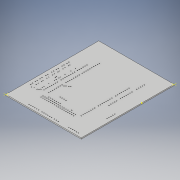
# Autodesk Inventor part: board
Saved by Autodesk Inventor 2019 (Build 230136000, 136)
## iProperties
Created: 2020-01-04
Part Number: board
Material: Типовые
Document SubType Name: Modeling
Designer: Петров Иван
Density: 1 g/cm^3
Appearance: По умолчанию
Author: Петров Иван
Autodesk Inventor part; units mm, degrees
ref_plane "YZ Plane" through (0, 0, 0) normal (1, 0, 0) x (0, 1, 0)
ref_plane "XZ Plane" through (0, 0, 0) normal (0, 1, 0) x (-1, 0, 0)
ref_plane "XY Plane" through (0, 0, 0) normal (0, 0, 1) x (1, 0, 0)
sketch "Эскиз1" plane through (0, 0, 0) normal (0, 1, 0) x (-1, 0, 0)
  circle A0 centre (25.4, 31.75) radius 0.508
  circle A1 centre (91.44, 17.78) radius 0.4064
  circle A2 centre (83.82, 45.72) radius 0.4064
  circle A3 centre (91.44, 45.72) radius 0.4064
  circle A4 centre (83.82, 3.81) radius 0.4064
  circle A5 centre (25.4, 39.37) radius 0.508
  circle A6 centre (25.4, 41.91) radius 0.508
  circle A7 centre (25.4, 44.45) radius 0.508
  circle A8 centre (25.4, 46.99) radius 0.508
  circle A9 centre (25.4, 49.53) radius 0.508
  circle A10 centre (25.4, 52.07) radius 0.508
  circle A11 centre (25.4, 54.61) radius 0.508
  circle A12 centre (25.4, 36.83) radius 0.508
  circle A13 centre (73.66, 34.29) radius 0.508
  circle A14 centre (73.66, 36.83) radius 0.508
  circle A15 centre (73.66, 39.37) radius 0.508
  circle A16 centre (73.66, 41.91) radius 0.508
  circle A17 centre (73.66, 44.45) radius 0.508
  circle A18 centre (73.66, 46.99) radius 0.508
  circle A19 centre (73.66, 49.53) radius 0.508
  circle A20 centre (73.66, 31.75) radius 0.508
  circle A21 centre (25.4, 16.51) radius 0.508
  circle A22 centre (25.4, 19.05) radius 0.508
  circle A23 centre (25.4, 21.59) radius 0.508
  circle A24 centre (25.4, 24.13) radius 0.508
  circle A25 centre (25.4, 26.67) radius 0.508
  circle A26 centre (25.4, 29.21) radius 0.508
  circle A27 centre (63.5, 57.15) radius 0.508
  circle A28 centre (25.4, 13.97) radius 0.508
  circle A29 centre (73.66, 11.43) radius 0.508
  circle A30 centre (73.66, 13.97) radius 0.508
  circle A31 centre (73.66, 16.51) radius 0.508
  circle A32 centre (73.66, 19.05) radius 0.508
  circle A33 centre (73.66, 21.59) radius 0.508
  circle A34 centre (73.66, 24.13) radius 0.508
  circle A35 centre (73.66, 26.67) radius 0.508
  circle A36 centre (73.66, 8.89) radius 0.508
  circle A37 centre (73.66, -10.16) radius 0.508
  circle A38 centre (73.66, -7.62) radius 0.508
  circle A39 centre (73.66, -5.08) radius 0.508
  circle A40 centre (73.66, -2.54) radius 0.508
  circle A41 centre (73.66, 0) radius 0.508
  circle A42 centre (73.66, 2.54) radius 0.508
  circle A43 centre (73.66, 5.08) radius 0.508
  circle A44 centre (73.66, -12.7) radius 0.508
  circle A45 centre (53.34, 59.69) radius 0.508
  circle A46 centre (53.34, 57.15) radius 0.508
  circle A47 centre (55.88, 59.69) radius 0.508
  circle A48 centre (55.88, 57.15) radius 0.508
  circle A49 centre (58.42, 59.69) radius 0.508
  circle A50 centre (58.42, 57.15) radius 0.508
  circle A51 centre (60.96, 59.69) radius 0.508
  circle A52 centre (60.96, 57.15) radius 0.508
  circle A53 centre (63.5, 59.69) radius 0.508
  circle A54 centre (91.44, 3.81) radius 0.4064
  circle A55 centre (66.04, 59.69) radius 0.508
  circle A56 centre (66.04, 57.15) radius 0.508
  circle A57 centre (68.58, 59.69) radius 0.508
  circle A58 centre (68.58, 57.15) radius 0.508
  circle A59 centre (71.12, 59.69) radius 0.508
  circle A60 centre (71.12, 57.15) radius 0.508
  circle A61 centre (33.02, 59.69) radius 0.508
  circle A62 centre (33.02, 57.15) radius 0.508
  circle A63 centre (35.56, 59.69) radius 0.508
  circle A64 centre (35.56, 57.15) radius 0.508
  circle A65 centre (38.1, 59.69) radius 0.508
  circle A66 centre (38.1, 57.15) radius 0.508
  circle A67 centre (40.64, 59.69) radius 0.508
  circle A68 centre (40.64, 57.15) radius 0.508
  circle A69 centre (43.18, 59.69) radius 0.508
  circle A70 centre (43.18, 57.15) radius 0.508
  circle A71 centre (45.72, 59.69) radius 0.508
  circle A72 centre (45.72, 57.15) radius 0.508
  circle A73 centre (48.26, 59.69) radius 0.508
  circle A74 centre (48.26, 57.15) radius 0.508
  circle A75 centre (50.8, 59.69) radius 0.508
  circle A76 centre (50.8, 57.15) radius 0.508
  circle A77 centre (30.48, 57.15) radius 0.508
  circle A78 centre (30.48, 59.69) radius 0.508
  circle A79 centre (73.66, 57.15) radius 0.508
  circle A80 centre (73.66, 59.69) radius 0.508
  circle A81 centre (25.4, -3.81) radius 0.508
  circle A82 centre (25.4, -1.27) radius 0.508
  circle A83 centre (25.4, 1.27) radius 0.508
  circle A84 centre (25.4, 3.81) radius 0.508
  circle A85 centre (25.4, 6.35) radius 0.508
  circle A86 centre (25.4, 8.89) radius 0.508
  circle A87 centre (73.66, -15.24) radius 0.508
  circle A88 centre (73.66, -17.78) radius 0.508
  circle A89 centre (25.4, -6.35) radius 0.508
  circle A90 centre (25.4, -8.89) radius 0.508
  circle A91 centre (20.32, 76.2) radius 0.508
  circle A92 centre (17.78, 76.2) radius 0.508
  circle A93 centre (15.24, 76.2) radius 0.508
  circle A94 centre (12.7, 76.2) radius 0.508
  circle A95 centre (10.16, 76.2) radius 0.508
  circle A96 centre (7.62, 76.2) radius 0.508
  circle A97 centre (55.88, 76.2) radius 0.508
  circle A98 centre (53.34, 76.2) radius 0.508
  circle A99 centre (50.8, 76.2) radius 0.508
  circle A100 centre (48.26, 76.2) radius 0.508
  circle A101 centre (45.72, 76.2) radius 0.508
  circle A102 centre (43.18, 76.2) radius 0.508
  circle A103 centre (73.152, 76.2) radius 0.508
  circle A104 centre (70.612, 76.2) radius 0.508
  circle A105 centre (68.072, 76.2) radius 0.508
  circle A106 centre (65.532, 76.2) radius 0.508
  circle A107 centre (62.992, 76.2) radius 0.508
  circle A108 centre (60.452, 76.2) radius 0.508
  circle A109 centre (5.08, 30.48) radius 0.508
  circle A110 centre (5.08, 33.02) radius 0.508
  circle A111 centre (5.08, 35.56) radius 0.508
  circle A112 centre (5.08, 38.1) radius 0.508
  circle A113 centre (5.08, 40.64) radius 0.508
  circle A114 centre (95.25, 15.24) radius 0.508
  circle A115 centre (95.25, 17.78) radius 0.508
  circle A116 centre (95.25, 36.83) radius 0.508
  circle A117 centre (95.25, 39.37) radius 0.508
  circle A118 centre (95.25, 1.27) radius 0.508
  circle A119 centre (95.25, 3.81) radius 0.508
  circle A120 centre (95.25, 21.59) radius 0.508
  circle A121 centre (95.25, 24.13) radius 0.508
  circle A122 centre (95.25, 29.21) radius 0.508
  circle A123 centre (95.25, 31.75) radius 0.508
  circle A124 centre (95.25, 43.18) radius 0.508
  circle A125 centre (95.25, 45.72) radius 0.508
  circle A126 centre (95.25, 49.53) radius 0.508
  circle A127 centre (95.25, 52.07) radius 0.508
  circle A128 centre (95.25, 7.62) radius 0.508
  circle A129 centre (95.25, 10.16) radius 0.508
  circle A130 centre (39.37, 76.2) radius 0.508
  circle A131 centre (36.83, 76.2) radius 0.508
  circle A132 centre (34.29, 76.2) radius 0.508
  circle A133 centre (19.05, 24.13) radius 0.508
  circle A134 centre (19.05, 21.59) radius 0.508
  circle A135 centre (19.05, 19.05) radius 0.508
  circle A136 centre (19.05, 16.51) radius 0.508
  circle A137 centre (19.05, 13.97) radius 0.508
  circle A138 centre (80.01, -7.62) radius 0.508
  circle A139 centre (80.01, -5.08) radius 0.508
  circle A140 centre (80.01, -2.54) radius 0.508
  circle A141 centre (80.01, 0) radius 0.508
  circle A142 centre (80.01, 2.54) radius 0.508
  circle A143 centre (80.01, 5.08) radius 0.508
  circle A144 centre (80.01, 8.89) radius 0.508
  circle A145 centre (80.01, 11.43) radius 0.508
  circle A146 centre (80.01, 13.97) radius 0.508
  circle A147 centre (80.01, 16.51) radius 0.508
  circle A148 centre (80.01, 19.05) radius 0.508
  circle A149 centre (80.01, 21.59) radius 0.508
  circle A150 centre (80.01, 24.13) radius 0.508
  circle A151 centre (80.01, 26.67) radius 0.508
  circle A152 centre (80.01, 31.75) radius 0.508
  circle A153 centre (80.01, 34.29) radius 0.508
  circle A154 centre (80.01, 36.83) radius 0.508
  circle A155 centre (80.01, 39.37) radius 0.508
  circle A156 centre (80.01, 41.91) radius 0.508
  circle A157 centre (80.01, 44.45) radius 0.508
  circle A158 centre (80.01, 46.99) radius 0.508
  circle A159 centre (80.01, 49.53) radius 0.508
  circle A160 centre (19.05, 8.89) radius 0.508
  circle A161 centre (19.05, 6.35) radius 0.508
  circle A162 centre (19.05, 3.81) radius 0.508
  circle A163 centre (19.05, 1.27) radius 0.508
  circle A164 centre (19.05, -1.27) radius 0.508
  circle A165 centre (19.05, -3.81) radius 0.508
  circle A166 centre (19.05, -6.35) radius 0.508
  circle A167 centre (19.05, -22.86) radius 0.508
  circle A168 centre (19.05, -20.32) radius 0.508
  circle A169 centre (19.05, -17.78) radius 0.508
  circle A170 centre (19.05, -15.24) radius 0.508
  circle A171 centre (19.05, -12.7) radius 0.508
  circle A172 centre (91.44, 10.16) radius 0.4064
  circle A173 centre (83.7929, 47.9789) radius 0.4064
  circle A174 centre (89.1811, 53.3671) radius 0.4064
  circle A175 centre (83.82, 24.13) radius 0.4064
  circle A176 centre (91.44, 24.13) radius 0.4064
  circle A177 centre (83.82, 10.16) radius 0.4064
  circle A178 centre (83.82, 39.37) radius 0.4064
  circle A179 centre (91.44, 39.37) radius 0.4064
  circle A180 centre (83.82, 31.75) radius 0.4064
  circle A181 centre (91.44, 31.75) radius 0.4064
  circle A182 centre (83.82, 17.78) radius 0.4064
  circle A183 centre (91.313, 19.685) radius 0.45
  circle A184 centre (68.58, 54.61) radius 0.5
  circle A185 centre (85.217, 53.467) radius 0.5
  circle A186 centre (55.88, 54.61) radius 0.5
  circle A187 centre (55.88, 46.99) radius 0.5
  circle A188 centre (67.31, 29.21) radius 0.5
  circle A189 centre (53.34, 54.61) radius 0.5
  circle A190 centre (53.34, 46.99) radius 0.5
  circle A191 centre (38.1, 54.61) radius 0.5
  circle A192 centre (83.82, 26.035) radius 0.5
  circle A193 centre (86.995, 26.035) radius 0.5
  circle A194 centre (66.04, 54.61) radius 0.5
  circle A195 centre (91.44, 5.588) radius 0.45
  circle A196 centre (91.44, 41.275) radius 0.45
  circle A197 centre (91.44, 54.61) radius 0.45
  circle A198 centre (91.44, 26.67) radius 0.45
  circle A199 centre (91.44, 48.26) radius 0.45
  circle A200 centre (91.44, 34.29) radius 0.45
  circle A201 centre (66.04, 27.94) radius 0.5
  circle A202 centre (91.44, 12.7) radius 0.45
  circle A203 centre (58.42, 54.61) radius 0.5
  circle A204 centre (58.42, 46.99) radius 0.5
  circle A205 centre (69.85, 30.48) radius 0.5
  circle A206 centre (86.614, 27.6726) radius 0.5
  circle A207 centre (83.947, 52.197) radius 0.5
  circle A208 centre (60.96, 54.61) radius 0.5
  circle A209 centre (60.96, 46.99) radius 0.5
  circle A210 centre (71.12, 31.75) radius 0.5
  circle A211 centre (83.82, 29.21) radius 0.5
  circle A212 centre (63.5, 54.61) radius 0.5
  circle A213 centre (82.677, 50.927) radius 0.5
  line L0 (100, 80) -> (0, 80)
  line L1 (0, 80) -> (0, -43.18)
  line L2 (0, -43.18) -> (100, -43.18)
  line L3 (100, -43.18) -> (100, 80)
  circle A214 centre (71.12, 59.69) radius 0.508
  line L4 (100, 80) -> (0, 80)
  line L5 (0, 80) -> (0, -43.18)
  line L6 (0, -43.18) -> (100, -43.18)
  line L7 (100, -43.18) -> (100, 80)
  point P0 (0, 0)
  constraints: 215 centre point, 16 end point, 2 parallel, 1 coincident, 1 concentric, 1 horizontal, 1 perpendicular
extrude "Выдавливание1" add sketch "Эскиз1" along normal blind 1.5
sketch "Эскиз2" plane through (0, 1.5, 0) normal (0, 1, 0) x (1, 0, 0)
  point P0 (0, 0)
  point P1 (0, 43.18)
  point P2 (-100, -80)
